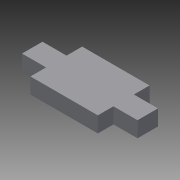
# Autodesk Inventor part: body-back
Saved by Autodesk Inventor 2013 (Build 170138000, 138)
## iProperties
Created: 2012-09-08
Part Number: body-back
Material: Generic
Document SubType Name: Modeling
Designer: frankenteddy
Density: 1 g/cm^3
Author: frankenteddy
Autodesk Inventor part; units mm, degrees
ref_plane "YZ Plane" through (0, 0, 0) normal (1, 0, 0) x (0, 1, 0)
ref_plane "XZ Plane" through (0, 0, 0) normal (0, 1, 0) x (-1, 0, 0)
ref_plane "XY Plane" through (0, 0, 0) normal (0, 0, 1) x (1, 0, 0)
sketch "Block1" plane through (0, 0, 0) normal (0, 0, 1) x (1, 0, 0)
  circle A0 centre (74.029, 24.2723) radius 1
  line L0 (49.279, 30.4723) -> (71.779, 30.4723)
  line L1 (71.779, 30.4723) -> (71.779, 18.0723)
  line L2 (71.779, 18.0723) -> (49.279, 18.0723)
  line L3 (49.279, 18.0723) -> (49.279, 30.4723)
  line L4 (49.279, 30.4723) -> (44.779, 30.4723)
  line L5 (44.779, 30.4723) -> (44.779, 18.0723)
  line L6 (44.779, 18.0723) -> (49.279, 18.0723)
  line L7 (49.279, 18.0723) -> (49.279, 30.4723)
  line L8 (71.779, 30.4723) -> (76.279, 30.4723)
  line L9 (76.279, 30.4723) -> (76.279, 18.0723)
  line L10 (76.279, 18.0723) -> (71.779, 18.0723)
  line L11 (71.779, 18.0723) -> (71.779, 30.4723)
  line L12 (44.779, 24.2723) -> (76.279, 24.2723) construction
  line L13 (47.029, 30.4723) -> (47.029, 18.0723) construction
  circle A1 centre (47.029, 24.2723) radius 1
  line L14 (74.029, 30.4723) -> (74.029, 18.0723) construction
  point P0 (60.979, 24.0984)
  dimension "d22" = 22.5
  dimension "d23" = 12.4
  dimension "d24" = 4.5
  dimension "d25" = 4.5
  dimension "d26" = 2
  dimension "d27" = 2
  measures "d22" distance of L1.end L2.end
  measures "d23" distance of L0.end L1.end
  measures "d24" distance of L6.end L5.end
  measures "d25" distance of L9.end L10.end
  measures "d26" diameter of A0
  measures "d27" diameter of A1
sketch "Sketch1" plane through (0, 0, 0) normal (0, 0, 1) x (1, 0, 0)
  line L0 (-92.7646, -8.503) -> (-89.7646, -8.503)
  line L1 (-89.7646, -8.503) -> (-89.7646, -11.753)
  line L2 (-89.7646, -11.753) -> (-92.7646, -11.753)
  line L3 (-92.7646, -11.753) -> (-92.7646, -8.503)
  line L4 (-92.7646, -21.6527) -> (-89.7646, -21.6527)
  line L5 (-89.7646, -21.6527) -> (-89.7646, -21.7527)
  line L6 (-89.7646, -21.7527) -> (-92.7646, -21.7527)
  line L7 (-92.7646, -21.7527) -> (-92.7646, -21.6527)
  line L8 (-39.1148, 14.5179) -> (-15.1148, 14.5179)
  line L9 (-15.1148, 14.5179) -> (-15.1148, 18.7679)
  line L10 (-15.1148, 18.7679) -> (-39.1148, 18.7679)
  line L11 (-39.1148, 18.7679) -> (-39.1148, 14.5179)
  line L12 (-34.1148, 22.0179) -> (-20.1148, 22.0179)
  line L13 (-20.1148, 22.0179) -> (-20.1148, 18.7679)
  line L14 (-20.1148, 18.7679) -> (-34.1148, 18.7679)
  line L15 (-34.1148, 18.7679) -> (-34.1148, 22.0179)
  line L16 (-39.1148, 16.6429) -> (-15.1148, 16.6429) construction
  line L17 (-27.1148, 22.0179) -> (-27.1148, 18.7679) construction
  line L18 (-27.1148, 18.7679) -> (-27.1148, 14.5179) construction
  line L19 (-34.1148, 11.2679) -> (-20.1148, 11.2679)
  line L20 (-20.1148, 11.2679) -> (-20.1148, 14.5179)
  line L21 (-20.1148, 14.5179) -> (-34.1148, 14.5179)
  line L22 (-34.1148, 14.5179) -> (-34.1148, 11.2679)
  line L23 (-27.1148, 11.2679) -> (-27.1148, 14.5179) construction
  point P0 (0, 0)
  point P1 (-27.1148, 14.5179)
  dimension "d3" = 3
  dimension "mat" = 3.25
  dimension "d5" = 3
  dimension "kerf" = 0.1
  dimension "d42" = 24
  dimension "d43" = 4.25
  dimension "d44" = 14
  dimension "d45" = 3.25
  constraints: 48 end point, 8 parallel, 7 symmetric about line, 6 midpoint, 4 horizontal, 4 perpendicular, 2 collinear
  measures "d3" distance of L1.end L2.end
  measures "mat" distance of L0.end L1.end
  measures "d5" distance of L5.end L6.end
  measures "kerf" distance of L4.end L5.end
  measures "d42" distance of L10.end L9.end
  measures "d43" distance of L9.end L8.end
  measures "d44" distance of L13.end L14.end
  measures "d45" distance of L12.end L13.end
extrude "Extrusion6" add sketch "Sketch1" along normal blind 3.25 contours L11 L10 L9 L8 | L8 L20 L19 L22 | L15 L12 L13 L10
equation "\"d45\" = mat"
equation "\"d46\" = mat"
body "Solid3"
